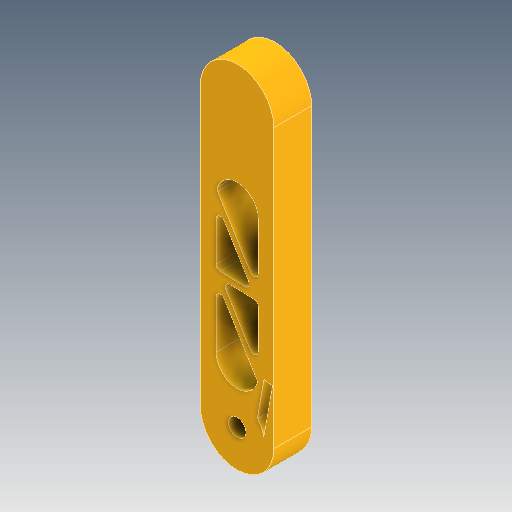
# Autodesk Inventor part: EslabonRodillaCadera
Saved by Autodesk Inventor 2021 (Build 250183000, 183)
## iProperties
Created: 2024-02-25
Part Number: EslabonRodillaCadera
Material: PLA
Document SubType Name: Modeling
Designer: Martin
Density: 1.27 g/cm^3
Appearance: PLA
Mass: 90.3407 g
Surface Area: 225.071 cm^2
Volume: 71.1344 cm^3
Author: Martin
Autodesk Inventor part; units mm, degrees
note: some values were not read from the file. Left out: dimensions or parameters whose unit could not be read.
ref_plane "YZ Plane" through (0, 0, 0) normal (1, 0, 0) x (0, 1, 0)
ref_plane "XZ Plane" through (0, 0, 0) normal (0, 1, 0) x (-1, 0, 0)
ref_plane "XY Plane" through (0, 0, 0) normal (0, 0, 1) x (1, 0, 0)
sketch "Sketch1" plane through (0, 0, 0) normal (0, 0, 1) x (1, 0, 0)
  line L0 (0.0065, 132.461) -> (0.0065, 0) construction
  line L1 (-17.4935, 132.461) -> (-17.4935, 0)
  line L2 (17.5065, 0) -> (17.5065, 132.461)
  arc A0 (17.5065, 132.461) -> (-17.4935, 132.461) centre (0.0065, 132.461) ccw
  arc A1 (-17.4935, 0) -> (17.5065, 0) centre (0.0065, 0) ccw
  circle A2 centre (0.0065, 0) radius 11.1
  circle A3 centre (0.0065, 131.961) radius 7.5
  line L3 (4.0065, 131.961) -> (4.0065, 109.961)
  line L4 (4.0065, 109.961) -> (-3.9935, 109.961)
  line L5 (-3.9935, 109.961) -> (-3.9935, 131.961)
  line L6 (-3.9935, 131.961) -> (4.0065, 131.961)
  line L7 (0.0065, 101.721) -> (0.0065, -30.5)
  line L8 (0.0065, 131.961) -> (5.7519, 127.1401)
  line L9 (0.0065, 131.961) -> (0.0065, 124.461) construction
  arc A4 (5.7519, 127.1401) -> (4.0065, 122.4546) centre (13.9526, 121.4175) ccw
  line L10 (0.0065, 131.961) -> (-5.7388, 127.1401)
  arc A5 (-3.9935, 122.4546) -> (-5.7388, 127.1401) centre (-13.9395, 121.4175) ccw
  line L11 (0.0065, 132.461) -> (0.0065, 108.461) construction
  line L12 (4.0065, 132.461) -> (4.0065, 108.461)
  line L13 (-3.9935, 108.461) -> (-3.9935, 132.461)
  arc A6 (4.0065, 132.461) -> (-3.9935, 132.461) centre (0.0065, 132.461) ccw
  arc A7 (-3.9935, 108.461) -> (4.0065, 108.461) centre (0.0065, 108.461) ccw
  point P0 (0.0065, 131.961)
  point P1 (-3.9935, 122.4546)
  point P2 (-5.7388, 127.1401)
  point P3 (0.0065, 120.461)
  point P4 (-3.9935, 109.961)
  point P5 (4.0065, 109.961)
  dimension "d38" = 15
  dimension "d19" = 35
  dimension "d20" = 22.2
  dimension "d39" = 22
  dimension "d40" = 8
  dimension "d41" = 4
  dimension "d42" = 4
  dimension "d43" = 50
  dimension "d44" = 5
  dimension "d45" = 10
  dimension "d50" = 24
  dimension "d59" = 132.461
  constraints: 32 end point, 12 point on circle, 8 tangent, 7 centre point, 4 parallel, 1 coincident, 1 equal length, 1 midpoint, 1 perpendicular, 1 point on line, 1 vertical, 3 other
  measures "d19" diameter of A1
  measures "d20" diameter of A2
  measures "d39" distance of L5.start L5.end
  measures "d40" distance of L3.end L5.start
  measures "d41" distance between parallel lines of L5 L7
  measures "d42" distance between parallel lines of L7 L3
  measures "d43" angle of L9 L8
  measures "d44" distance of L8.end A4.end
  measures "d45" radius of A4
  measures "d50" distance of L11.start L11.end
  measures "d59" distance of L0.end L0.start
extrude "Extrusion1" add sketch "Sketch1" along normal mid plane 6
sketch "Sketch6" plane through (0, 0, 3) normal (0, 0, 1) x (1, 0, 0)
  arc A0 (-17.4935, 0) -> (17.5065, 0) centre (0.0065, 0) ccw projected
  line L0 (17.5065, 0) -> (17.5065, 132.461) projected
  arc A1 (17.5065, 132.461) -> (-17.4935, 132.461) centre (0.0065, 132.461) ccw projected
  line L1 (-17.4935, 132.461) -> (-17.4935, 0) projected
  arc A2 (-3.9935, 108.461) -> (4.0065, 108.461) centre (0.0065, 108.461) ccw projected
  line L2 (-3.9935, 108.461) -> (-3.9935, 122.4546) projected
  arc A3 (-3.9935, 122.4546) -> (-5.7388, 127.1401) centre (-13.9395, 121.4175) ccw projected
  arc A4 (5.7519, 127.1401) -> (-5.7388, 127.1401) centre (0.0065, 131.961) ccw projected
  arc A5 (5.7519, 127.1401) -> (4.0065, 122.4546) centre (13.9526, 121.4175) ccw projected
  line L3 (4.0065, 122.4546) -> (4.0065, 108.461) projected
  circle A6 centre (0.0065, 0) radius 11.1 projected
  point P0 (0, 0)
extrude "Extrusion4" add sketch "Sketch6" along normal blind 2 contours L1 A1 L0 A0 | L2 A3 A4 A5 L3 A2
sketch "Sketch7" plane through (0, 0, 5) normal (0, 0, 1) x (1, 0, 0)
  line L0 (0, 244.3) -> (0, -244.3) projected
  line L1 (17.5065, 0) -> (17.5065, 132.461) projected
  arc A0 (17.5065, 132.461) -> (-17.4935, 132.461) centre (0.0065, 132.461) ccw projected
  line L2 (-17.4935, 132.461) -> (-17.4935, 0) projected
  arc A1 (-17.4935, 0) -> (17.5065, 0) centre (0.0065, 0) ccw projected
  circle A2 centre (0.0065, 0) radius 11.1 projected
  circle A3 centre (0.0065, 0) radius 4.1
  point P0 (0, 0)
  point P1 (0, 11.1)
  point P2 (0, -11.1)
  point P3 (0, -17.5)
  point P4 (0, 149.961)
  dimension "d53" = 8.2
  constraints: 1 centre point, 1 coincident
  measures "d53" diameter of A3
extrude "Extrusion5" add sketch "Sketch7" along normal blind 10 contours A0 L1 A1 L0 A2 | L0 A2 A1 L2 A0 | A2 L0 A3 | L0 A3 A2
sketch "Sketch9" plane through (0, 0, -3) normal (0, 0, -1) x (-1, 0, 0)
  line L0 (-4.0065, 122.4546) -> (-4.0065, 108.461) projected
  arc A0 (-4.0065, 108.461) -> (3.9935, 108.461) centre (-0.0065, 108.461) ccw projected
  line L1 (3.9935, 108.461) -> (3.9935, 122.4546) projected
  arc A1 (5.7388, 127.1401) -> (3.9935, 122.4546) centre (13.9395, 121.4175) ccw projected
  arc A2 (5.7388, 127.1401) -> (-5.7519, 127.1401) centre (-0.0065, 131.961) ccw projected
  arc A3 (-4.0065, 122.4546) -> (-5.7519, 127.1401) centre (-13.9526, 121.4175) ccw projected
  line L2 (4.1935, 122.4442) -> (4.1935, 108.461)
  arc A4 (-4.2065, 108.461) -> (4.1935, 108.461) centre (-0.0065, 108.461) ccw
  line L3 (-4.2065, 108.461) -> (-4.2065, 122.4442)
  arc A5 (-4.2065, 122.4442) -> (-5.9109, 127.0184) centre (-13.9526, 121.4175) ccw
  arc A6 (5.8978, 127.0184) -> (-5.9109, 127.0184) centre (-0.0065, 131.961) ccw
  arc A7 (5.8978, 127.0184) -> (4.1935, 122.4442) centre (13.9395, 121.4175) ccw
  point P0 (0, 0)
  dimension "d60" = 0.2
  constraints: 8 point on circle, 4 centre point, 4 end point, 5 other
  measures "d60" radial gap between concentric circles of A1 A7
extrude "Extrusion7" cut sketch "Sketch9" against normal up to surface (6 mm away)
sketch "Sketch11" plane through (0, 0, 15) normal (0, 0, 1) x (1, 0, 0)
  line L0 (10.9002, -1.9232) -> (15.7624, 25.6515)
  line L1 (10.9002, -1.9232) -> (38.9002, -1.9232) construction
  circle A0 centre (-0.0065, 0) radius 11.075
  circle A1 centre (-0.0065, 0) radius 12
  line L2 (16.7472, 25.4778) -> (12.092, -0.9232)
  line L3 (12.8079, 26.1724) -> (7.325, -4.9232)
  circle A2 centre (-0.0065, 0) radius 13
  circle A3 centre (-0.0065, 0) radius 10
  line L4 (12.8079, 26.1724) -> (16.7472, 25.4778)
  point P0 (0, 0)
  point P1 (0, 0)
  point P2 (9.7149, 8.631)
  point P3 (12.7213, 2.6461)
  dimension "d74" = 28
  dimension "d75" = 80
  dimension "d76" = 24
  dimension "d77" = 1
  dimension "d78" = 3
  dimension "d80" = 2
  constraints: 10 end point, 3 centre point, 1 coincident, 1 equal length, 1 horizontal, 4 other
  measures "d74" distance of L0.start L0.end
  measures "d75" angle of L1 L0
  measures "d76" diameter of A1
  measures "d77" distance between parallel lines of L0 L2
  measures "d78" distance between parallel lines of L0 L3
  measures "d80" radial gap between concentric circles of A1 A3
extrude "Extrusion10" cut sketch "Sketch11" against normal blind 8 contours A2 L3 L4 L0 | L0 L4 L2 A2
sketch "Sketch13" plane through (0, 0, -3) normal (0, 0, -1) x (-1, 0, 0)
  line L0 (0, 101.0671) -> (0, 16.0671) construction
  line L1 (-10, 91.0671) -> (-10, 26.0671)
  line L2 (10, 26.0671) -> (10, 91.0671)
  arc A0 (10, 91.0671) -> (-10, 91.0671) centre (0, 91.0671) ccw
  arc A1 (-10, 26.0671) -> (10, 26.0671) centre (0, 26.0671) ccw
  line L3 (10, 26.0671) -> (10, 58.9004)
  line L4 (-10, 91.0671) -> (-10, 58.2338)
  line L5 (-10, 26.0671) -> (10, 58.9004)
  line L6 (10, 58.9004) -> (-10, 58.2338)
  line L7 (-10, 58.2338) -> (10, 91.0671)
  line L8 (33.0369, 58.1675) -> (-10, 56.7329)
  line L9 (32.9369, 61.1658) -> (-10.05, 59.7329)
  line L10 (-8.719, 57.4534) -> (11.281, 90.2868)
  line L11 (-11.281, 59.0141) -> (9.7071, 93.4696)
  line L12 (-9.7071, 23.6646) -> (11.281, 58.1201)
  line L13 (-11.281, 26.8474) -> (8.719, 59.6808)
  point P0 (0, 0)
  point P1 (0, 58.5671)
  point P2 (39.2224, 129.4846)
  point P3 (-10, 61.1171)
  point P4 (-10, 107.6003)
  point P5 (7.2741, 57.3087)
  point P6 (-10, 28.9505)
  point P7 (10, 56.017)
  point P8 (10, 60.4013)
  point P9 (-7.2741, 59.8255)
  point P10 (10, 88.1837)
  dimension "d97" = 20
  dimension "d98" = 65
  dimension "d99" = 32.8333
  dimension "d100" = 32.8333
  dimension "d101" = 1.5
  dimension "d102" = 1.5
  dimension "d103" = 1.5
  dimension "d104" = 1.5
  dimension "d105" = 1.5
  dimension "d106" = 1.5
  constraints: 30 end point, 8 point on circle, 7 parallel, 5 point on line, 4 tangent, 2 centre point, 1 midpoint, 1 vertical
  measures "d97" diameter of A1
  measures "d98" distance of A0.centre A1.centre
  measures "d99" distance of L2.start L3.end
  measures "d100" distance of L1.start L4.end
  measures "d101" distance between parallel lines of L6 L8
  measures "d102" distance between parallel lines of L6 L9
  measures "d103" distance between parallel lines of L7 L10
  measures "d104" distance between parallel lines of L7 L11
  measures "d105" distance between parallel lines of L5 L12
  measures "d106" distance between parallel lines of L5 L13
extrude "Extrusion12" cut sketch "Sketch13" against normal up to next contours L8 L13 L1 | L1 A0 L11 | L10 L2 L9 | L12 L2 A1
fillet "Fillet2" radius 2 10 edges at (-9.7071, 93.4696, 6) (-10, 88.1837, 6) (10, 28.9505, 6) (10, 61.1171, 6) (-7.2741, 57.3087, 6) (-10, 56.017, 6) (9.7071, 23.6646, 6) (-10, 60.4013, 6) (7.2741, 59.8255, 6) (10, 56.7329, 6)
move or copy body "Move1" bodies to move or copy 1 copy no translate (0, -131.75, 0)
move or copy body "Move2" bodies to move or copy 1 copy no translate (0, 0, -6)
body "Solid1"
